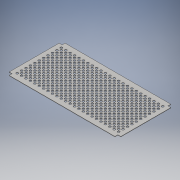
# Autodesk Inventor part: BellyPan Aluminium
Saved by Autodesk Inventor 2016 (Build 200138000, 138)
## iProperties
Created: 2018-05-06
Part Number: BellyPan Aluminium
Material: Generic
Document SubType Name: Sheet Metal
Designer: Kade
Density: 1 g/cm^3
Sheet Metal Rule: Default
Appearance: Default
Author: Kade
Autodesk Inventor part; units mm, degrees
ref_plane "YZ Plane" through (0, 0, 0) normal (1, 0, 0) x (0, 1, 0)
ref_plane "XZ Plane" through (0, 0, 0) normal (0, 1, 0) x (-1, 0, 0)
ref_plane "XY Plane" through (0, 0, 0) normal (0, 0, 1) x (1, 0, 0)
sketch "Sketch1" plane through (0, 0, 0) normal (0, 1, 0) x (-1, 0, 0)
  line L0 (-457.2, 241.3) -> (457.2, 241.3)
  line L1 (482.6, 215.9) -> (482.6, -215.9)
  line L2 (457.2, -241.3) -> (-457.2, -241.3)
  line L3 (-482.6, -215.9) -> (-482.6, 215.9)
  line L4 (-457.2, 215.9) -> (457.2, 215.9)
  line L5 (457.2, 215.9) -> (457.2, -215.9)
  line L6 (457.2, -215.9) -> (-457.2, -215.9)
  line L7 (-457.2, -215.9) -> (-457.2, 215.9)
  line L8 (-457.2, 215.9) -> (457.2, -215.9) construction
  line L9 (457.2, 215.9) -> (-457.2, -215.9) construction
  line L10 (457.2, -215.9) -> (482.6, -215.9)
  line L11 (457.2, -241.3) -> (457.2, -215.9)
  line L12 (457.2, 241.3) -> (457.2, 215.9)
  line L13 (457.2, 215.9) -> (482.6, 215.9)
  line L14 (-457.2, 241.3) -> (-457.2, 215.9)
  line L15 (-457.2, 215.9) -> (-482.6, 215.9)
  line L16 (-457.2, -241.3) -> (-457.2, -215.9)
  line L17 (-457.2, -215.9) -> (-482.6, -215.9)
  circle A0 centre (438.15, 190.5) radius 9.525
  circle A1 centre (419.1, 171.45) radius 9.525
  circle A2 centre (438.15, 152.4) radius 9.525
  circle A3 centre (438.15, 114.3) radius 9.525
  circle A4 centre (438.15, 76.2) radius 9.525
  circle A5 centre (438.15, 38.1) radius 9.525
  circle A6 centre (438.15, 0) radius 9.525
  circle A7 centre (438.15, -38.1) radius 9.525
  circle A8 centre (438.15, -76.2) radius 9.525
  circle A9 centre (438.15, -114.3) radius 9.525
  circle A10 centre (438.15, -152.4) radius 9.525
  circle A11 centre (438.15, -190.5) radius 9.525
  circle A12 centre (400.05, 190.5) radius 9.525
  circle A13 centre (400.05, 152.4) radius 9.525
  circle A14 centre (400.05, 114.3) radius 9.525
  circle A15 centre (400.05, 76.2) radius 9.525
  circle A16 centre (400.05, 38.1) radius 9.525
  circle A17 centre (400.05, 0) radius 9.525
  circle A18 centre (400.05, -38.1) radius 9.525
  circle A19 centre (400.05, -76.2) radius 9.525
  circle A20 centre (400.05, -114.3) radius 9.525
  circle A21 centre (400.05, -152.4) radius 9.525
  circle A22 centre (400.05, -190.5) radius 9.525
  circle A23 centre (361.95, 190.5) radius 9.525
  circle A24 centre (361.95, 152.4) radius 9.525
  circle A25 centre (361.95, 114.3) radius 9.525
  circle A26 centre (361.95, 76.2) radius 9.525
  circle A27 centre (361.95, 38.1) radius 9.525
  circle A28 centre (361.95, 0) radius 9.525
  circle A29 centre (361.95, -38.1) radius 9.525
  circle A30 centre (361.95, -76.2) radius 9.525
  circle A31 centre (361.95, -114.3) radius 9.525
  circle A32 centre (361.95, -152.4) radius 9.525
  circle A33 centre (361.95, -190.5) radius 9.525
  circle A34 centre (323.85, 190.5) radius 9.525
  circle A35 centre (323.85, 152.4) radius 9.525
  circle A36 centre (323.85, 114.3) radius 9.525
  circle A37 centre (323.85, 76.2) radius 9.525
  circle A38 centre (323.85, 38.1) radius 9.525
  circle A39 centre (323.85, 0) radius 9.525
  circle A40 centre (323.85, -38.1) radius 9.525
  circle A41 centre (323.85, -76.2) radius 9.525
  circle A42 centre (323.85, -114.3) radius 9.525
  circle A43 centre (323.85, -152.4) radius 9.525
  circle A44 centre (323.85, -190.5) radius 9.525
  circle A45 centre (285.75, 190.5) radius 9.525
  circle A46 centre (285.75, 152.4) radius 9.525
  circle A47 centre (285.75, 114.3) radius 9.525
  circle A48 centre (285.75, 76.2) radius 9.525
  circle A49 centre (285.75, 38.1) radius 9.525
  circle A50 centre (285.75, 0) radius 9.525
  circle A51 centre (285.75, -38.1) radius 9.525
  circle A52 centre (285.75, -76.2) radius 9.525
  circle A53 centre (285.75, -114.3) radius 9.525
  circle A54 centre (285.75, -152.4) radius 9.525
  circle A55 centre (285.75, -190.5) radius 9.525
  circle A56 centre (247.65, 190.5) radius 9.525
  circle A57 centre (247.65, 152.4) radius 9.525
  circle A58 centre (247.65, 114.3) radius 9.525
  circle A59 centre (247.65, 76.2) radius 9.525
  circle A60 centre (247.65, 38.1) radius 9.525
  circle A61 centre (247.65, 0) radius 9.525
  circle A62 centre (247.65, -38.1) radius 9.525
  circle A63 centre (247.65, -76.2) radius 9.525
  circle A64 centre (247.65, -114.3) radius 9.525
  circle A65 centre (247.65, -152.4) radius 9.525
  circle A66 centre (247.65, -190.5) radius 9.525
  circle A67 centre (209.55, 190.5) radius 9.525
  circle A68 centre (209.55, 152.4) radius 9.525
  circle A69 centre (209.55, 114.3) radius 9.525
  circle A70 centre (209.55, 76.2) radius 9.525
  circle A71 centre (209.55, 38.1) radius 9.525
  circle A72 centre (209.55, 0) radius 9.525
  circle A73 centre (209.55, -38.1) radius 9.525
  circle A74 centre (209.55, -76.2) radius 9.525
  circle A75 centre (209.55, -114.3) radius 9.525
  circle A76 centre (209.55, -152.4) radius 9.525
  circle A77 centre (209.55, -190.5) radius 9.525
  circle A78 centre (171.45, 190.5) radius 9.525
  circle A79 centre (171.45, 152.4) radius 9.525
  circle A80 centre (171.45, 114.3) radius 9.525
  circle A81 centre (171.45, 76.2) radius 9.525
  circle A82 centre (171.45, 38.1) radius 9.525
  circle A83 centre (171.45, 0) radius 9.525
  circle A84 centre (171.45, -38.1) radius 9.525
  circle A85 centre (171.45, -76.2) radius 9.525
  circle A86 centre (171.45, -114.3) radius 9.525
  circle A87 centre (171.45, -152.4) radius 9.525
  circle A88 centre (171.45, -190.5) radius 9.525
  circle A89 centre (133.35, 190.5) radius 9.525
  circle A90 centre (133.35, 152.4) radius 9.525
  circle A91 centre (133.35, 114.3) radius 9.525
  circle A92 centre (133.35, 76.2) radius 9.525
  circle A93 centre (133.35, 38.1) radius 9.525
  circle A94 centre (133.35, 0) radius 9.525
  circle A95 centre (133.35, -38.1) radius 9.525
  circle A96 centre (133.35, -76.2) radius 9.525
  circle A97 centre (133.35, -114.3) radius 9.525
  circle A98 centre (133.35, -152.4) radius 9.525
  circle A99 centre (133.35, -190.5) radius 9.525
  circle A100 centre (95.25, 190.5) radius 9.525
  circle A101 centre (95.25, 152.4) radius 9.525
  circle A102 centre (95.25, 114.3) radius 9.525
  circle A103 centre (95.25, 76.2) radius 9.525
  circle A104 centre (95.25, 38.1) radius 9.525
  circle A105 centre (95.25, 0) radius 9.525
  circle A106 centre (95.25, -38.1) radius 9.525
  circle A107 centre (95.25, -76.2) radius 9.525
  circle A108 centre (95.25, -114.3) radius 9.525
  circle A109 centre (95.25, -152.4) radius 9.525
  circle A110 centre (95.25, -190.5) radius 9.525
  circle A111 centre (57.15, 190.5) radius 9.525
  circle A112 centre (57.15, 152.4) radius 9.525
  circle A113 centre (57.15, 114.3) radius 9.525
  circle A114 centre (57.15, 76.2) radius 9.525
  circle A115 centre (57.15, 38.1) radius 9.525
  circle A116 centre (57.15, 0) radius 9.525
  circle A117 centre (57.15, -38.1) radius 9.525
  circle A118 centre (57.15, -76.2) radius 9.525
  circle A119 centre (57.15, -114.3) radius 9.525
  circle A120 centre (57.15, -152.4) radius 9.525
  circle A121 centre (57.15, -190.5) radius 9.525
  circle A122 centre (19.05, 190.5) radius 9.525
  circle A123 centre (19.05, 152.4) radius 9.525
  circle A124 centre (19.05, 114.3) radius 9.525
  circle A125 centre (19.05, 76.2) radius 9.525
  circle A126 centre (19.05, 38.1) radius 9.525
  circle A127 centre (19.05, 0) radius 9.525
  circle A128 centre (19.05, -38.1) radius 9.525
  circle A129 centre (19.05, -76.2) radius 9.525
  circle A130 centre (19.05, -114.3) radius 9.525
  circle A131 centre (19.05, -152.4) radius 9.525
  circle A132 centre (19.05, -190.5) radius 9.525
  circle A133 centre (-19.05, 190.5) radius 9.525
  circle A134 centre (-19.05, 152.4) radius 9.525
  circle A135 centre (-19.05, 114.3) radius 9.525
  circle A136 centre (-19.05, 76.2) radius 9.525
  circle A137 centre (-19.05, 38.1) radius 9.525
  circle A138 centre (-19.05, 0) radius 9.525
  circle A139 centre (-19.05, -38.1) radius 9.525
  circle A140 centre (-19.05, -76.2) radius 9.525
  circle A141 centre (-19.05, -114.3) radius 9.525
  circle A142 centre (-19.05, -152.4) radius 9.525
  circle A143 centre (-19.05, -190.5) radius 9.525
  circle A144 centre (-57.15, 190.5) radius 9.525
  circle A145 centre (-57.15, 152.4) radius 9.525
  circle A146 centre (-57.15, 114.3) radius 9.525
  circle A147 centre (-57.15, 76.2) radius 9.525
  circle A148 centre (-57.15, 38.1) radius 9.525
  circle A149 centre (-57.15, 0) radius 9.525
  circle A150 centre (-57.15, -38.1) radius 9.525
  circle A151 centre (-57.15, -76.2) radius 9.525
  circle A152 centre (-57.15, -114.3) radius 9.525
  circle A153 centre (-57.15, -152.4) radius 9.525
  circle A154 centre (-57.15, -190.5) radius 9.525
  circle A155 centre (-95.25, 190.5) radius 9.525
  circle A156 centre (-95.25, 152.4) radius 9.525
  circle A157 centre (-95.25, 114.3) radius 9.525
  circle A158 centre (-95.25, 76.2) radius 9.525
  circle A159 centre (-95.25, 38.1) radius 9.525
  circle A160 centre (-95.25, 0) radius 9.525
  circle A161 centre (-95.25, -38.1) radius 9.525
  circle A162 centre (-95.25, -76.2) radius 9.525
  circle A163 centre (-95.25, -114.3) radius 9.525
  circle A164 centre (-95.25, -152.4) radius 9.525
  circle A165 centre (-95.25, -190.5) radius 9.525
  circle A166 centre (-133.35, 190.5) radius 9.525
  circle A167 centre (-133.35, 152.4) radius 9.525
  circle A168 centre (-133.35, 114.3) radius 9.525
  circle A169 centre (-133.35, 76.2) radius 9.525
  circle A170 centre (-133.35, 38.1) radius 9.525
  circle A171 centre (-133.35, 0) radius 9.525
  circle A172 centre (-133.35, -38.1) radius 9.525
  circle A173 centre (-133.35, -76.2) radius 9.525
  circle A174 centre (-133.35, -114.3) radius 9.525
  circle A175 centre (-133.35, -152.4) radius 9.525
  circle A176 centre (-133.35, -190.5) radius 9.525
  circle A177 centre (-171.45, 190.5) radius 9.525
  circle A178 centre (-171.45, 152.4) radius 9.525
  circle A179 centre (-171.45, 114.3) radius 9.525
  circle A180 centre (-171.45, 76.2) radius 9.525
  circle A181 centre (-171.45, 38.1) radius 9.525
  circle A182 centre (-171.45, 0) radius 9.525
  circle A183 centre (-171.45, -38.1) radius 9.525
  circle A184 centre (-171.45, -76.2) radius 9.525
  circle A185 centre (-171.45, -114.3) radius 9.525
  circle A186 centre (-171.45, -152.4) radius 9.525
  circle A187 centre (-171.45, -190.5) radius 9.525
  circle A188 centre (-209.55, 190.5) radius 9.525
  circle A189 centre (-209.55, 152.4) radius 9.525
  circle A190 centre (-209.55, 114.3) radius 9.525
  circle A191 centre (-209.55, 76.2) radius 9.525
  circle A192 centre (-209.55, 38.1) radius 9.525
  circle A193 centre (-209.55, 0) radius 9.525
  circle A194 centre (-209.55, -38.1) radius 9.525
  circle A195 centre (-209.55, -76.2) radius 9.525
  circle A196 centre (-209.55, -114.3) radius 9.525
  circle A197 centre (-209.55, -152.4) radius 9.525
  circle A198 centre (-209.55, -190.5) radius 9.525
  circle A199 centre (-247.65, 190.5) radius 9.525
  circle A200 centre (-247.65, 152.4) radius 9.525
  circle A201 centre (-247.65, 114.3) radius 9.525
  circle A202 centre (-247.65, 76.2) radius 9.525
  circle A203 centre (-247.65, 38.1) radius 9.525
  circle A204 centre (-247.65, 0) radius 9.525
  circle A205 centre (-247.65, -38.1) radius 9.525
  circle A206 centre (-247.65, -76.2) radius 9.525
  circle A207 centre (-247.65, -114.3) radius 9.525
  circle A208 centre (-247.65, -152.4) radius 9.525
  circle A209 centre (-247.65, -190.5) radius 9.525
  circle A210 centre (-285.75, 190.5) radius 9.525
  circle A211 centre (-285.75, 152.4) radius 9.525
  circle A212 centre (-285.75, 114.3) radius 9.525
  circle A213 centre (-285.75, 76.2) radius 9.525
  circle A214 centre (-285.75, 38.1) radius 9.525
  circle A215 centre (-285.75, 0) radius 9.525
  circle A216 centre (-285.75, -38.1) radius 9.525
  circle A217 centre (-285.75, -76.2) radius 9.525
  circle A218 centre (-285.75, -114.3) radius 9.525
  circle A219 centre (-285.75, -152.4) radius 9.525
  circle A220 centre (-285.75, -190.5) radius 9.525
  circle A221 centre (-323.85, 190.5) radius 9.525
  circle A222 centre (-323.85, 152.4) radius 9.525
  circle A223 centre (-323.85, 114.3) radius 9.525
  circle A224 centre (-323.85, 76.2) radius 9.525
  circle A225 centre (-323.85, 38.1) radius 9.525
  circle A226 centre (-323.85, 0) radius 9.525
  circle A227 centre (-323.85, -38.1) radius 9.525
  circle A228 centre (-323.85, -76.2) radius 9.525
  circle A229 centre (-323.85, -114.3) radius 9.525
  circle A230 centre (-323.85, -152.4) radius 9.525
  circle A231 centre (-323.85, -190.5) radius 9.525
  circle A232 centre (-361.95, 190.5) radius 9.525
  circle A233 centre (-361.95, 152.4) radius 9.525
  circle A234 centre (-361.95, 114.3) radius 9.525
  circle A235 centre (-361.95, 76.2) radius 9.525
  circle A236 centre (-361.95, 38.1) radius 9.525
  circle A237 centre (-361.95, 0) radius 9.525
  circle A238 centre (-361.95, -38.1) radius 9.525
  circle A239 centre (-361.95, -76.2) radius 9.525
  circle A240 centre (-361.95, -114.3) radius 9.525
  circle A241 centre (-361.95, -152.4) radius 9.525
  circle A242 centre (-361.95, -190.5) radius 9.525
  circle A243 centre (-400.05, 190.5) radius 9.525
  circle A244 centre (-400.05, 152.4) radius 9.525
  circle A245 centre (-400.05, 114.3) radius 9.525
  circle A246 centre (-400.05, 76.2) radius 9.525
  circle A247 centre (-400.05, 38.1) radius 9.525
  circle A248 centre (-400.05, 0) radius 9.525
  circle A249 centre (-400.05, -38.1) radius 9.525
  circle A250 centre (-400.05, -76.2) radius 9.525
  circle A251 centre (-400.05, -114.3) radius 9.525
  circle A252 centre (-400.05, -152.4) radius 9.525
  circle A253 centre (-400.05, -190.5) radius 9.525
  circle A254 centre (-438.15, 190.5) radius 9.525
  circle A255 centre (-438.15, 152.4) radius 9.525
  circle A256 centre (-438.15, 114.3) radius 9.525
  circle A257 centre (-438.15, 76.2) radius 9.525
  circle A258 centre (-438.15, 38.1) radius 9.525
  circle A259 centre (-438.15, 0) radius 9.525
  circle A260 centre (-438.15, -38.1) radius 9.525
  circle A261 centre (-438.15, -76.2) radius 9.525
  circle A262 centre (-438.15, -114.3) radius 9.525
  circle A263 centre (-438.15, -152.4) radius 9.525
  circle A264 centre (-438.15, -190.5) radius 9.525
  circle A265 centre (419.1, 133.35) radius 9.525
  circle A266 centre (419.1, 95.25) radius 9.525
  circle A267 centre (419.1, 57.15) radius 9.525
  circle A268 centre (419.1, 19.05) radius 9.525
  circle A269 centre (419.1, -19.05) radius 9.525
  circle A270 centre (419.1, -57.15) radius 9.525
  circle A271 centre (419.1, -95.25) radius 9.525
  circle A272 centre (419.1, -133.35) radius 9.525
  circle A273 centre (419.1, -171.45) radius 9.525
  circle A274 centre (381, 171.45) radius 9.525
  circle A275 centre (381, 133.35) radius 9.525
  circle A276 centre (381, 95.25) radius 9.525
  circle A277 centre (381, 57.15) radius 9.525
  circle A278 centre (381, 19.05) radius 9.525
  circle A279 centre (381, -19.05) radius 9.525
  circle A280 centre (381, -57.15) radius 9.525
  circle A281 centre (381, -95.25) radius 9.525
  circle A282 centre (381, -133.35) radius 9.525
  circle A283 centre (381, -171.45) radius 9.525
  circle A284 centre (342.9, 171.45) radius 9.525
  circle A285 centre (342.9, 133.35) radius 9.525
  circle A286 centre (342.9, 95.25) radius 9.525
  circle A287 centre (342.9, 57.15) radius 9.525
  circle A288 centre (342.9, 19.05) radius 9.525
  circle A289 centre (342.9, -19.05) radius 9.525
  circle A290 centre (342.9, -57.15) radius 9.525
  circle A291 centre (342.9, -95.25) radius 9.525
  circle A292 centre (342.9, -133.35) radius 9.525
  circle A293 centre (342.9, -171.45) radius 9.525
  circle A294 centre (304.8, 171.45) radius 9.525
  circle A295 centre (304.8, 133.35) radius 9.525
  circle A296 centre (304.8, 95.25) radius 9.525
  circle A297 centre (304.8, 57.15) radius 9.525
  circle A298 centre (304.8, 19.05) radius 9.525
  circle A299 centre (304.8, -19.05) radius 9.525
  circle A300 centre (304.8, -57.15) radius 9.525
  circle A301 centre (304.8, -95.25) radius 9.525
  circle A302 centre (304.8, -133.35) radius 9.525
  circle A303 centre (304.8, -171.45) radius 9.525
  circle A304 centre (266.7, 171.45) radius 9.525
  circle A305 centre (266.7, 133.35) radius 9.525
  circle A306 centre (266.7, 95.25) radius 9.525
  circle A307 centre (266.7, 57.15) radius 9.525
  circle A308 centre (266.7, 19.05) radius 9.525
  circle A309 centre (266.7, -19.05) radius 9.525
  circle A310 centre (266.7, -57.15) radius 9.525
  circle A311 centre (266.7, -95.25) radius 9.525
  circle A312 centre (266.7, -133.35) radius 9.525
  circle A313 centre (266.7, -171.45) radius 9.525
  circle A314 centre (228.6, 171.45) radius 9.525
  circle A315 centre (228.6, 133.35) radius 9.525
  circle A316 centre (228.6, 95.25) radius 9.525
  circle A317 centre (228.6, 57.15) radius 9.525
  circle A318 centre (228.6, 19.05) radius 9.525
  circle A319 centre (228.6, -19.05) radius 9.525
  circle A320 centre (228.6, -57.15) radius 9.525
  circle A321 centre (228.6, -95.25) radius 9.525
  circle A322 centre (228.6, -133.35) radius 9.525
  circle A323 centre (228.6, -171.45) radius 9.525
  circle A324 centre (190.5, 171.45) radius 9.525
  circle A325 centre (190.5, 133.35) radius 9.525
  circle A326 centre (190.5, 95.25) radius 9.525
  circle A327 centre (190.5, 57.15) radius 9.525
  circle A328 centre (190.5, 19.05) radius 9.525
  circle A329 centre (190.5, -19.05) radius 9.525
  circle A330 centre (190.5, -57.15) radius 9.525
  circle A331 centre (190.5, -95.25) radius 9.525
  circle A332 centre (190.5, -133.35) radius 9.525
  circle A333 centre (190.5, -171.45) radius 9.525
  circle A334 centre (152.4, 171.45) radius 9.525
  circle A335 centre (152.4, 133.35) radius 9.525
  circle A336 centre (152.4, 95.25) radius 9.525
  circle A337 centre (152.4, 57.15) radius 9.525
  circle A338 centre (152.4, 19.05) radius 9.525
  circle A339 centre (152.4, -19.05) radius 9.525
  circle A340 centre (152.4, -57.15) radius 9.525
  circle A341 centre (152.4, -95.25) radius 9.525
  circle A342 centre (152.4, -133.35) radius 9.525
  circle A343 centre (152.4, -171.45) radius 9.525
  circle A344 centre (114.3, 171.45) radius 9.525
  circle A345 centre (114.3, 133.35) radius 9.525
  circle A346 centre (114.3, 95.25) radius 9.525
  circle A347 centre (114.3, 57.15) radius 9.525
  circle A348 centre (114.3, 19.05) radius 9.525
  circle A349 centre (114.3, -19.05) radius 9.525
  circle A350 centre (114.3, -57.15) radius 9.525
  circle A351 centre (114.3, -95.25) radius 9.525
  circle A352 centre (114.3, -133.35) radius 9.525
  circle A353 centre (114.3, -171.45) radius 9.525
  circle A354 centre (76.2, 171.45) radius 9.525
  circle A355 centre (76.2, 133.35) radius 9.525
  circle A356 centre (76.2, 95.25) radius 9.525
  circle A357 centre (76.2, 57.15) radius 9.525
  circle A358 centre (76.2, 19.05) radius 9.525
  circle A359 centre (76.2, -19.05) radius 9.525
  circle A360 centre (76.2, -57.15) radius 9.525
  circle A361 centre (76.2, -95.25) radius 9.525
  circle A362 centre (76.2, -133.35) radius 9.525
  circle A363 centre (76.2, -171.45) radius 9.525
  circle A364 centre (38.1, 171.45) radius 9.525
  circle A365 centre (38.1, 133.35) radius 9.525
  circle A366 centre (38.1, 95.25) radius 9.525
  circle A367 centre (38.1, 57.15) radius 9.525
  circle A368 centre (38.1, 19.05) radius 9.525
  circle A369 centre (38.1, -19.05) radius 9.525
  circle A370 centre (38.1, -57.15) radius 9.525
  circle A371 centre (38.1, -95.25) radius 9.525
  circle A372 centre (38.1, -133.35) radius 9.525
  circle A373 centre (38.1, -171.45) radius 9.525
  circle A374 centre (0, 171.45) radius 9.525
  circle A375 centre (0, 133.35) radius 9.525
  circle A376 centre (0, 95.25) radius 9.525
  circle A377 centre (0, 57.15) radius 9.525
  circle A378 centre (0, 19.05) radius 9.525
  circle A379 centre (0, -19.05) radius 9.525
  circle A380 centre (0, -57.15) radius 9.525
  circle A381 centre (0, -95.25) radius 9.525
  circle A382 centre (0, -133.35) radius 9.525
  circle A383 centre (0, -171.45) radius 9.525
  circle A384 centre (-38.1, 171.45) radius 9.525
  circle A385 centre (-38.1, 133.35) radius 9.525
  circle A386 centre (-38.1, 95.25) radius 9.525
  circle A387 centre (-38.1, 57.15) radius 9.525
  circle A388 centre (-38.1, 19.05) radius 9.525
  circle A389 centre (-38.1, -19.05) radius 9.525
  circle A390 centre (-38.1, -57.15) radius 9.525
  circle A391 centre (-38.1, -95.25) radius 9.525
  circle A392 centre (-38.1, -133.35) radius 9.525
  circle A393 centre (-38.1, -171.45) radius 9.525
  circle A394 centre (-76.2, 171.45) radius 9.525
  circle A395 centre (-76.2, 133.35) radius 9.525
  circle A396 centre (-76.2, 95.25) radius 9.525
  circle A397 centre (-76.2, 57.15) radius 9.525
  circle A398 centre (-76.2, 19.05) radius 9.525
  circle A399 centre (-76.2, -19.05) radius 9.525
  circle A400 centre (-76.2, -57.15) radius 9.525
  circle A401 centre (-76.2, -95.25) radius 9.525
  circle A402 centre (-76.2, -133.35) radius 9.525
  circle A403 centre (-76.2, -171.45) radius 9.525
  circle A404 centre (-114.3, 171.45) radius 9.525
  circle A405 centre (-114.3, 133.35) radius 9.525
  circle A406 centre (-114.3, 95.25) radius 9.525
  circle A407 centre (-114.3, 57.15) radius 9.525
  circle A408 centre (-114.3, 19.05) radius 9.525
  circle A409 centre (-114.3, -19.05) radius 9.525
  circle A410 centre (-114.3, -57.15) radius 9.525
  circle A411 centre (-114.3, -95.25) radius 9.525
  circle A412 centre (-114.3, -133.35) radius 9.525
  circle A413 centre (-114.3, -171.45) radius 9.525
  circle A414 centre (-152.4, 171.45) radius 9.525
  circle A415 centre (-152.4, 133.35) radius 9.525
  circle A416 centre (-152.4, 95.25) radius 9.525
  circle A417 centre (-152.4, 57.15) radius 9.525
  circle A418 centre (-152.4, 19.05) radius 9.525
  circle A419 centre (-152.4, -19.05) radius 9.525
  circle A420 centre (-152.4, -57.15) radius 9.525
  circle A421 centre (-152.4, -95.25) radius 9.525
  circle A422 centre (-152.4, -133.35) radius 9.525
  circle A423 centre (-152.4, -171.45) radius 9.525
  circle A424 centre (-190.5, 171.45) radius 9.525
  circle A425 centre (-190.5, 133.35) radius 9.525
  circle A426 centre (-190.5, 95.25) radius 9.525
  circle A427 centre (-190.5, 57.15) radius 9.525
  circle A428 centre (-190.5, 19.05) radius 9.525
  circle A429 centre (-190.5, -19.05) radius 9.525
  circle A430 centre (-190.5, -57.15) radius 9.525
  circle A431 centre (-190.5, -95.25) radius 9.525
  circle A432 centre (-190.5, -133.35) radius 9.525
  circle A433 centre (-190.5, -171.45) radius 9.525
  circle A434 centre (-228.6, 171.45) radius 9.525
  circle A435 centre (-228.6, 133.35) radius 9.525
  circle A436 centre (-228.6, 95.25) radius 9.525
  circle A437 centre (-228.6, 57.15) radius 9.525
  circle A438 centre (-228.6, 19.05) radius 9.525
  circle A439 centre (-228.6, -19.05) radius 9.525
  circle A440 centre (-228.6, -57.15) radius 9.525
  circle A441 centre (-228.6, -95.25) radius 9.525
  circle A442 centre (-228.6, -133.35) radius 9.525
  circle A443 centre (-228.6, -171.45) radius 9.525
  circle A444 centre (-266.7, 171.45) radius 9.525
  circle A445 centre (-266.7, 133.35) radius 9.525
  circle A446 centre (-266.7, 95.25) radius 9.525
  circle A447 centre (-266.7, 57.15) radius 9.525
  circle A448 centre (-266.7, 19.05) radius 9.525
  circle A449 centre (-266.7, -19.05) radius 9.525
  circle A450 centre (-266.7, -57.15) radius 9.525
  circle A451 centre (-266.7, -95.25) radius 9.525
  circle A452 centre (-266.7, -133.35) radius 9.525
  circle A453 centre (-266.7, -171.45) radius 9.525
  circle A454 centre (-304.8, 171.45) radius 9.525
  circle A455 centre (-304.8, 133.35) radius 9.525
  circle A456 centre (-304.8, 95.25) radius 9.525
  circle A457 centre (-304.8, 57.15) radius 9.525
  circle A458 centre (-304.8, 19.05) radius 9.525
  circle A459 centre (-304.8, -19.05) radius 9.525
  circle A460 centre (-304.8, -57.15) radius 9.525
  circle A461 centre (-304.8, -95.25) radius 9.525
  circle A462 centre (-304.8, -133.35) radius 9.525
  circle A463 centre (-304.8, -171.45) radius 9.525
  circle A464 centre (-342.9, 171.45) radius 9.525
  circle A465 centre (-342.9, 133.35) radius 9.525
  circle A466 centre (-342.9, 95.25) radius 9.525
  circle A467 centre (-342.9, 57.15) radius 9.525
  circle A468 centre (-342.9, 19.05) radius 9.525
  circle A469 centre (-342.9, -19.05) radius 9.525
  circle A470 centre (-342.9, -57.15) radius 9.525
  circle A471 centre (-342.9, -95.25) radius 9.525
  circle A472 centre (-342.9, -133.35) radius 9.525
  circle A473 centre (-342.9, -171.45) radius 9.525
  circle A474 centre (-381, 171.45) radius 9.525
  circle A475 centre (-381, 133.35) radius 9.525
  circle A476 centre (-381, 95.25) radius 9.525
  circle A477 centre (-381, 57.15) radius 9.525
  circle A478 centre (-381, 19.05) radius 9.525
  circle A479 centre (-381, -19.05) radius 9.525
  circle A480 centre (-381, -57.15) radius 9.525
  circle A481 centre (-381, -95.25) radius 9.525
  circle A482 centre (-381, -133.35) radius 9.525
  circle A483 centre (-381, -171.45) radius 9.525
  circle A484 centre (-419.1, 171.45) radius 9.525
  circle A485 centre (-419.1, 133.35) radius 9.525
  circle A486 centre (-419.1, 95.25) radius 9.525
  circle A487 centre (-419.1, 57.15) radius 9.525
  circle A488 centre (-419.1, 19.05) radius 9.525
  circle A489 centre (-419.1, -19.05) radius 9.525
  circle A490 centre (-419.1, -57.15) radius 9.525
  circle A491 centre (-419.1, -95.25) radius 9.525
  circle A492 centre (-419.1, -133.35) radius 9.525
  circle A493 centre (-419.1, -171.45) radius 9.525
  point P0 (0, 0)
  dimension "d2" = 914.4
  dimension "d3" = 431.8
  dimension "d4" = 965.2
  dimension "d5" = 482.6
  dimension "d6" = 25.4
  dimension "d7" = 25.4
  dimension "d8" = 25.4
  dimension "d9" = 25.4
  dimension "d10" = 25.4
  dimension "d11" = 25.4
  dimension "d12" = 25.4
  dimension "d13" = 25.4
  dimension "d14" = 25.4
  dimension "d15" = 19.05
  dimension "d16" = 25.4
  dimension "d17" = 19.05
  dimension "d18" = 19.05
  dimension "d19" = 19.05
  dimension "d20" = 19.05
  dimension "d23" = 38.1
  dimension "d26" = 38.1
  dimension "d31" = 38.1
  dimension "d34" = 38.1
  constraints: 494 centre point, 36 end point, 5 horizontal, 4 parallel, 2 midpoint, 2 perpendicular, 2 vertical, 984 other
  measures "d2" distance of L5.end L6.end
  measures "d3" distance of L4.end L5.end
  measures "d4" distance between parallel lines of L3 L1
  measures "d5" distance between parallel lines of L0 L2
  measures "d6" distance between parallel lines of L5 L1
  measures "d7" distance between parallel lines of L6 L2
  measures "d8" distance of L2.end L6.end
  measures "d9" distance of L6.end L3.start
  measures "d10" distance of L0.start L4.start
  measures "d11" distance of L4.start L3.end
  measures "d12" distance of L4.end L1.start
  measures "d13" distance of L0.end L4.end
  measures "d14" distance of L2.start L5.end
  measures "d15" diameter of A0
  measures "d16" distance from line of L4 A0.centre
  measures "d17" distance from line of L5 A0.centre
  measures "d18" diameter of A1
  measures "d19" horizontal distance of A0.centre A1.centre
  measures "d20" horizontal distance of A0.centre A1.centre
  measures "d23" distance of A0.centre A2.centre
  measures "d26" distance of A0.centre A12.centre
  measures "d31" distance of A1.centre A265.centre
  measures "d34" distance of A1.centre A274.centre
extrude "Extrusion1" add sketch "Sketch1" along normal blind 3.175
equation "\"BendRadius\" = Thickness"
equation "\"BendReliefWidth\" = Thickness"
equation "\"BendReliefDepth\" = 0.5 * Thickness"
equation "\"CornerReliefSize\" = 4 * Thickness"
equation "\"MinimumRemnant\" = 2 * Thickness"
equation "\"TransitionRadius\" = BendRadius"
equation "\"JacobiRadiusSize\" = BendRadius"
equation "\"GapSize\" = Thickness"
equation "\"Thickness\" = 3.048"
body "Solid1"
